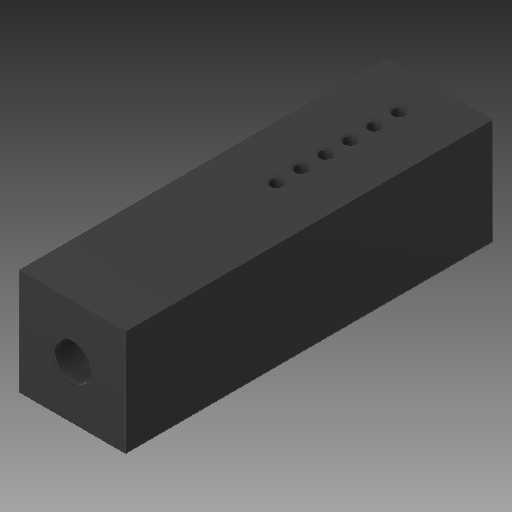
# Autodesk Inventor part: male_long_part2_9_2018
Saved by Autodesk Inventor 2019 (Build 230136000, 136)
## iProperties
Created: 2018-09-06
Part Number: male_long_part2_9_2018
Material: Acetal Resin, Black
Document SubType Name: Sheet Metal
Designer: FiolkaLab
Density: 1.425 g/cm^3
Sheet Metal Rule: Default_mm
Appearance: Smooth - Black
Author: FiolkaLab
Autodesk Inventor part; units mm, degrees
ref_plane "YZ Plane" through (0, 0, 0) normal (1, 0, 0) x (0, 1, 0)
ref_plane "XZ Plane" through (0, 0, 0) normal (0, 1, 0) x (-1, 0, 0)
ref_plane "XY Plane" through (0, 0, 0) normal (0, 0, 1) x (1, 0, 0)
sketch "Sketch1" plane through (0, 0, 0) normal (0, 0, 1) x (1, 0, 0)
  line L0 (0, 0) -> (13, 0)
  line L1 (13, 0) -> (13, 13)
  line L2 (13, 13) -> (0, 13)
  line L3 (0, 13) -> (0, 0)
  dimension "d0" = 13
  dimension "d1" = 13
  constraints: 8 end point, 2 parallel, 1 horizontal, 1 perpendicular
  measures "d0" distance of L2.end L1.end
  measures "d1" distance of L1.end L0.end
extrude "Extrusion1" add sketch "Sketch1" along normal blind 45
sketch "Sketch2" plane through (0, 0, 0) normal (0, 0, -1) x (-1, 0, 0)
  circle A0 centre (-6.5, 6.5) radius 3.75
  line L0 (0, 13) -> (0, 0) projected
  line L1 (0, 0) -> (-13, 0) projected
  dimension "d4" = 7.5
  dimension "d5" = 6.5
  dimension "d6" = 6.5
  constraints: 1 centre point
  measures "d4" diameter of A0
  measures "d5" distance from line of A0.centre L0
  measures "d6" distance from line of L1 A0.centre
hole "Hole1" at (6.5, 6.5, 0) direction (0, 0, 1) diameter 4.5 end through all counterbore diameter 7.5 counterbore depth 40.5
sketch "Sketch3" plane through (0, 0, 0) normal (0, -1, 0) x (1, 0, 0)
  circle A0 centre (6.5, 5) radius 1
  line L0 (13, 0) -> (13, 45) projected
  line L1 (0, 0) -> (13, 0) projected
  circle A1 centre (6.5, 8) radius 1
  circle A2 centre (6.5, 11) radius 1
  circle A3 centre (6.5, 14) radius 1
  circle A4 centre (6.5, 17) radius 1
  circle A5 centre (6.5, 20) radius 1
  dimension "d14" = 2
  dimension "d15" = 6.5
  dimension "d16" = 5
  dimension "d17" = 2
  dimension "d18" = 3
  dimension "d19" = 6.5
  dimension "d20" = 2
  dimension "d21" = 3
  dimension "d22" = 6.5
  dimension "d23" = 2
  dimension "d24" = 3
  dimension "d25" = 6.5
  dimension "d26" = 2
  dimension "d27" = 3
  dimension "d28" = 2
  dimension "d29" = 3
  dimension "d30" = 6.5
  constraints: 6 centre point
  measures "d14" diameter of A0
  measures "d15" distance from line of A0.centre L0
  measures "d16" distance from line of L1 A0.centre
  measures "d17" diameter of A1
  measures "d18" distance of A0.centre A1.centre
  measures "d19" distance from line of L0 A1.centre
  measures "d20" diameter of A2
  measures "d21" distance of A1.centre A2.centre
  measures "d22" distance from line of L0 A2.centre
  measures "d23" diameter of A3
  measures "d24" distance of A2.centre A3.centre
  measures "d25" distance from line of L0 A3.centre
  measures "d26" diameter of A4
  measures "d27" distance of A3.centre A4.centre
  measures "d28" diameter of A5
  measures "d29" distance of A4.centre A5.centre
  measures "d30" distance from line of L0 A5.centre
hole "Hole2" at (6.5, 0, 5) at (6.5, 0, 8) at (6.5, 0, 11) at (6.5, 0, 14) at (6.5, 0, 17) at (6.5, 0, 20) direction (0, 1, 0) diameter 1.5 end through all
equation "\"d12\" = Thickness"
equation "\"d36\" = Thickness"
equation "\"BendRadius\" = Thickness"
equation "\"BendReliefWidth\" = Thickness"
equation "\"BendReliefDepth\" = 0.5 * Thickness"
equation "\"CornerReliefSize\" = 4 * Thickness"
equation "\"MinimumRemnant\" = 2 * Thickness"
equation "\"TransitionRadius\" = BendRadius"
equation "\"JacobiRadiusSize\" = BendRadius"
equation "\"GapSize\" = Thickness"
equation "\"Thickness\" = 0.5"
body "Solid1"
